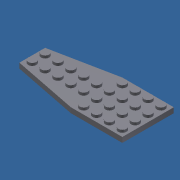
# Autodesk Inventor part: LEGO Brick 2413
Saved by Autodesk Inventor 2011 SP2 (Build 150309200, 309)
## iProperties
Created: 2011-09-28
Part Number: LEGO Brick 2413
Cost Center: 0 kg
Material: Steel
Document SubType Name: Modeling
Designer: BvH
Authority: 0 mm^3
Stock Number: =<Filenr>_<Document number>
Density: 7.85 g/cm^3
Company: Allseas Engineering BV
Subject: =<Title><TITLE 1_2> <TITLE 2_2>
Author: BvH
Act. Code: DW000
SaveDate: 2011-07-28
SaveTime: 18:32
FileName: Standard
TotalMass: 0 kg
TotalVolume: 0 mm^3
Autodesk Inventor part; units mm, degrees
ref_plane "YZ Plane" through (0, 0, 0) normal (1, 0, 0) x (0, 1, 0)
ref_plane "XZ Plane" through (0, 0, 0) normal (0, 1, 0) x (-1, 0, 0)
ref_plane "XY Plane" through (0, 0, 0) normal (0, 0, 1) x (1, 0, 0)
sketch "Sketch1" plane through (0, 0, 0) normal (0, 0, 1) x (1, 0, 0)
  line L0 (-36, 16) -> (36, 16)
  line L1 (36, 16) -> (36, -16)
  line L2 (36, -16) -> (-36, -16)
  line L3 (-36, -16) -> (-36, 16)
  line L4 (-36, -16) -> (36, 16) construction
  line L5 (4, 16) -> (-36, 8)
  line L6 (-36, -8) -> (4, -16)
  line L7 (4, 16) -> (4, -16) construction
  circle A0 centre (-32, 4) radius 2.5
  circle A1 centre (32, 12) radius 2.5
  point P0 (0, 0)
  point P1 (0, 0)
  dimension "d0" = 32
  dimension "d1" = 72
  dimension "d2" = 32
  dimension "d3" = 16
  dimension "d4" = 5
  dimension "d5" = 4
  dimension "d6" = 4
  dimension "d7" = 4
  dimension "d8" = 4
  constraints: 16 end point, 4 point on line, 3 vertical, 2 centre point, 2 horizontal, 1 coincident, 1 equal length, 1 equal radius, 1 midpoint
  measures "d0" distance between parallel lines of L2 L0
  measures "d1" distance between parallel lines of L3 L1
  measures "d2" distance between parallel lines of L1 L7
  measures "d3" distance of L6.start L5.end
  measures "d4" diameter of A0
  measures "d5" distance from line of L1 A1.centre
  measures "d6" distance from line of A1.centre L0
  measures "d7" distance from line of A0.centre L3
  measures "d8" horizontal distance of A0.centre L5.end
extrude "Extrusion1" add sketch "Sketch1" against normal blind 3.2 contours L0 L1 L2 L6 L3 L5 | A0 | A1
extrude "Extrusion2" add sketch "Sketch1" along normal blind 1.6 contours A0
pattern_linear "Rectangular Pattern1" count 5 spacing 8 along (1, 0, 0) count 2 spacing 8 along (0, -1, 0) of "Extrusion2"
extrude "Extrusion3" add sketch "Sketch1" along normal blind 1.6 contours A1
pattern_linear "Rectangular Pattern2" count 4 spacing 8 along (-1, 0, 0) count 4 spacing 8 along (0, -1, 0) of "Extrusion3"
sketch "Sketch2" plane through (0, 0, -3.2) normal (0, 0, -1) x (-1, 0, 0)
  circle A0 centre (32, 4) radius 2.5 construction
  circle A1 centre (24, 4) radius 2.5 construction
  circle A2 centre (16, 4) radius 2.5 construction
  circle A3 centre (8, 4) radius 2.5 construction
  circle A4 centre (0, 4) radius 2.5 construction
  circle A5 centre (-8, 4) radius 2.5 construction
  circle A6 centre (-16, 4) radius 2.5 construction
  circle A7 centre (-24, 4) radius 2.5 construction
  circle A8 centre (-32, 4) radius 2.5 construction
  circle A9 centre (-32, 12) radius 2.5 construction
  circle A10 centre (-24, 12) radius 2.5 construction
  circle A11 centre (-16, 12) radius 2.5 construction
  circle A12 centre (-8, 12) radius 2.5 construction
  circle A13 centre (-32, -4) radius 2.5 construction
  circle A14 centre (-24, -4) radius 2.5 construction
  circle A15 centre (-16, -4) radius 2.5 construction
  circle A16 centre (-8, -4) radius 2.5 construction
  circle A17 centre (0, -4) radius 2.5 construction
  circle A18 centre (8, -4) radius 2.5 construction
  circle A19 centre (16, -4) radius 2.5 construction
  circle A20 centre (24, -4) radius 2.5 construction
  circle A21 centre (32, -4) radius 2.5 construction
  circle A22 centre (-8, -12) radius 2.5 construction
  circle A23 centre (-16, -12) radius 2.5 construction
  circle A24 centre (-24, -12) radius 2.5 construction
  circle A25 centre (-32, -12) radius 2.5 construction
  line L0 (-34.5, -14.5) -> (-5.5, -14.5)
  line L1 (-5.5, -14.5) -> (-5.5, -6.5)
  line L2 (-5.5, -6.5) -> (34.5, -6.5)
  line L3 (34.5, -6.5) -> (34.5, 6.5)
  line L4 (34.5, 6.5) -> (-5.5, 6.5)
  line L5 (-5.5, 6.5) -> (-5.5, 14.5)
  line L6 (-5.5, 14.5) -> (-34.5, 14.5)
  line L7 (-34.5, 14.5) -> (-34.5, -14.5)
  circle A26 centre (-28, -8) radius 3.1569
  circle A27 centre (-28, -8) radius 2.3569
  circle A28 centre (-28, 0) radius 3.1569
  circle A29 centre (-28, 0) radius 2.3569
  dimension "d27" = 0.8
  constraints: 16 end point, 13 tangent, 4 centre point, 4 horizontal, 4 vertical, 2 coincident, 2 equal radius
  measures "d27" radial gap between concentric circles of A26 A27
extrude "Extrusion4" cut sketch "Sketch2" against normal blind 2 contours L7 L6 L5 L4 L3 L2 L1 L0 | A26 | A27 | A28 | A29
extrude "Extrusion5" add sketch "Sketch2" against normal blind 2 contours A26
extrude "Extrusion6" add sketch "Sketch2" against normal blind 2 contours A28
pattern_linear "Rectangular Pattern3" count 3 spacing 8 along (-1, 0, 0) count 2 spacing 16 along (0, 1, 0) of "Extrusion5"
pattern_linear "Rectangular Pattern4" count 8 spacing 8 along (-1, 0, 0) of "Extrusion6"
body "Solid1"
